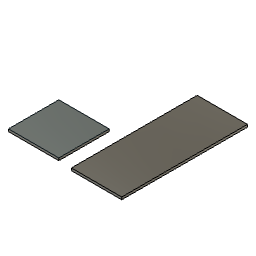
platform (Autodesk Fusion 360 design; units mm, degrees)
Autodesk Fusion 360 part; units mm, degrees
sketch "Sketch1" plane through (0, 0, 0) normal (0, 0, 1) x (1, 0, 0)
  line L0 (0, 0) -> (0, 200)
  line L1 (0, 0) -> (80, 0)
  line L2 (80, 0) -> (80, 200)
  line L3 (80, 200) -> (0, 200)
  dimension "d1" = 200
  dimension "d2" = 80
  constraint coincident L0.start L1.start
  constraint vertical L0
  constraint perpendicular L0 L1
  constraint perpendicular L1 L2
  constraint perpendicular L0 L3
  measures "d1" distance of L0.start L0.end
  measures "d2" distance of L0.end L2.end
extrude "Extrude1" add sketch "Sketch1" along normal blind 3.8 makes body 1
sketch "Sketch2" plane through (0, 0, 3.8) normal (0, 0, 1) x (-1, 0, 0)
  line L0 (0, 0) -> (-80, 0)
  line L1 (-80, 0) -> (-80, -200)
  line L2 (-80, -200) -> (0, -200)
  line L3 (0, -200) -> (0, 0)
  line L4 (100, 0) -> (100, -80)
  line L5 (100, -80) -> (20, -80)
  line L6 (20, -80) -> (20, 0)
  line L7 (20, 0) -> (100, 0)
  constraint vertical L4
  constraint perpendicular L4 L5
  constraint perpendicular L5 L6
  constraint perpendicular L4 L7
extrude "Extrude2" add sketch "Sketch2" along normal blind 3.8 separate body contours L4 L5 L6 L7 makes body 2
sketch "Sketch3" plane through (0, 0, 7.6) normal (0, 0, 1) x (-1, 0, 0)
  line L0 (20, 0) -> (20, -80)
  line L1 (20, -80) -> (100, -80)
  line L2 (100, -80) -> (100, 0)
  line L3 (100, 0) -> (20, 0)
